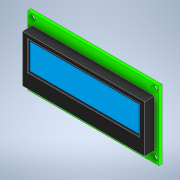
# Autodesk Inventor part: Adafruit_2675
Saved by Autodesk Inventor 2021 (Build 250183000, 183)
## iProperties
Created: 2020-11-05
Part Number: Adafruit_2675
Material: Generic
Document SubType Name: Modeling
Designer: Viktor
Density: 1 g/cm^3
Appearance: Default
Author: Viktor
Autodesk Inventor part; units mm, degrees
ref_plane "YZ Plane" through (0, 0, 0) normal (1, 0, 0) x (0, 1, 0)
ref_plane "XZ Plane" through (0, 0, 0) normal (0, 1, 0) x (-1, 0, 0)
ref_plane "XY Plane" through (0, 0, 0) normal (0, 0, 1) x (1, 0, 0)
sketch "Sketch1" plane through (0, 0, 0) normal (0, 0, 1) x (1, 0, 0)
  line L0 (-33.25, -17.5) -> (33.25, -17.5)
  line L1 (33.25, -17.5) -> (33.25, 17.5)
  line L2 (33.25, 17.5) -> (-33.25, 17.5)
  line L3 (-33.25, 17.5) -> (-33.25, -17.5)
  line L4 (-33.25, -17.5) -> (33.25, 17.5) construction
  line L5 (33.25, -17.5) -> (-33.25, 17.5) construction
  point P0 (0, 0)
  dimension "d0" = 66.5
  dimension "d1" = 35
  constraints: 12 end point, 2 midpoint, 2 parallel, 1 horizontal, 1 perpendicular
  measures "d0" distance of L1.end L2.end
  measures "d1" distance of L0.end L1.end
extrude "Extrusion1" add sketch "Sketch1" along normal blind 1.6
sketch "Sketch2" plane through (0, 0, 1.6) normal (0, 0, 1) x (1, 0, 0)
  line L0 (-46.55, 0) -> (46.55, 0) construction
  line L1 (0, -24.5) -> (0, 24.5) construction
  circle A0 centre (-31.05, 15.3) radius 1.6
  line L2 (33.25, 17.5) -> (-33.25, 17.5) construction
  line L3 (-33.25, 17.5) -> (-33.25, -17.5) construction
  circle A1 centre (31.05, 15.3) radius 1.6
  circle A2 centre (-31.05, -15.3) radius 1.6
  line L4 (33.25, -17.5) -> (-33.25, -17.5) construction
  circle A3 centre (31.05, -15.3) radius 1.6
  point P0 (0, 0)
  dimension "d4" = 3.2
  dimension "d5" = 0.6
  dimension "d6" = 0.6
  constraints: 4 centre point, 4 symmetric about line, 2 end point, 3 other
  measures "d4" diameter of A0
  measures "d5" distance edge to line of A0 L2
  measures "d6" distance edge to line of A0 L3
extrude "Extrusion2" cut sketch "Sketch2" against normal through all
sketch "Sketch3" plane through (0, 0, 1.6) normal (0, 0, 1) x (1, 0, 0)
  line L0 (0, 24.5) -> (0, -24.5) projected
  line L1 (-31, -12) -> (31, -12)
  line L2 (31, -12) -> (31, 12)
  line L3 (31, 12) -> (-31, 12)
  line L4 (-31, 12) -> (-31, -12)
  line L5 (-31, -12) -> (31, 12) construction
  line L6 (31, -12) -> (-31, 12) construction
  point P0 (0, 0)
  dimension "d9" = 24
  dimension "d10" = 62
  constraints: 12 end point, 2 midpoint, 2 parallel, 1 horizontal, 1 perpendicular
  measures "d9" distance of L3.end L1.start
  measures "d10" distance of L2.end L3.end
extrude "Extrusion3" add sketch "Sketch3" along normal blind 5 separate body
sketch "Sketch4" plane through (0, 0, 6.6) normal (0, 0, 1) x (1, 0, 0)
  line L0 (0, -24.5) -> (0, 24.5) projected
  line L1 (-28.5, -5) -> (28.5, -5)
  line L2 (28.5, -5) -> (28.5, 10)
  line L3 (28.5, 10) -> (-28.5, 10)
  line L4 (-28.5, 10) -> (-28.5, -5)
  line L5 (-28.5, -5) -> (28.5, 10) construction
  line L6 (28.5, -5) -> (-28.5, 10) construction
  line L7 (31, 12) -> (-31, 12) projected
  point P0 (0, 0)
  point P1 (0, 2.5)
  dimension "d13" = 15
  dimension "d14" = 57
  dimension "d15" = 2
  constraints: 12 end point, 2 midpoint, 2 parallel, 1 horizontal, 1 perpendicular, 1 point on line
  measures "d13" distance of L3.end L1.start
  measures "d14" distance of L2.end L3.end
  measures "d15" distance between parallel lines of L7 L3
extrude "Extrusion4" cut sketch "Sketch4" against normal blind 0.5 bodies 2
sketch "Sketch5" plane through (0, 0, 6.1) normal (0, 0, 1) x (1, 0, 0)
  line L0 (0, 24.5) -> (0, -24.5) projected
  line L1 (-27.5, -4.1) -> (27.5, -4.1)
  line L2 (27.5, -4.1) -> (27.5, 9)
  line L3 (27.5, 9) -> (-27.5, 9)
  line L4 (-27.5, 9) -> (-27.5, -4.1)
  line L5 (-27.5, -4.1) -> (27.5, 9) construction
  line L6 (27.5, -4.1) -> (-27.5, 9) construction
  line L7 (31, 12) -> (-31, 12) projected
  point P0 (0, 0)
  point P1 (0, 2.45)
  dimension "d18" = 13.1
  dimension "d19" = 55
  dimension "d20" = 3
  constraints: 12 end point, 2 midpoint, 2 parallel, 1 horizontal, 1 perpendicular, 1 point on line
  measures "d18" distance of L3.end L1.start
  measures "d19" distance of L2.end L3.end
  measures "d20" distance between parallel lines of L7 L3
extrude "Extrusion5" cut sketch "Sketch5" against normal blind 0.5 bodies 2
sketch "Sketch6" plane through (0, 0, 5.6) normal (0, 0, 1) x (1, 0, 0)
  line L0 (27.5, -4.1) -> (-27.5, -4.1) projected
  line L1 (27.5, 9) -> (27.5, -4.1) projected
  line L2 (-27.5, 9) -> (27.5, 9) projected
  line L3 (-27.5, -4.1) -> (-27.5, 9) projected
  point P0 (0, 0)
extrude "Extrusion6" add sketch "Sketch6" along normal blind 0.5 separate body
sketch "Sketch7" plane through (0, 0, 6.6) normal (0, 0, 1) x (1, 0, 0)
  circle A0 centre (0, 0) radius 6.7082
  constraints: 1 centre point, 1 coincident
equation "\"d6\" = d5"
body "Solid1"
body "Solid2"
body "Solid3"
